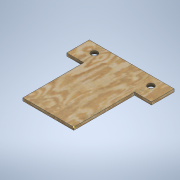
# Autodesk Inventor part: shooter bottom
Saved by Autodesk Inventor 2020 (Build 240168000, 168)
## iProperties
Created: 2020-01-27
Part Number: shooter bottom
Material: Wood (Oak)
Document SubType Name: Modeling
Designer: 1cikaychapman
Density: 0.76 g/cm^3
Appearance: Plywood - Weathered
Author: 1cikaychapman
Autodesk Inventor part; units mm, degrees
ref_plane "YZ Plane" through (0, 0, 0) normal (1, 0, 0) x (0, 1, 0)
ref_plane "XZ Plane" through (0, 0, 0) normal (0, 1, 0) x (-1, 0, 0)
ref_plane "XY Plane" through (0, 0, 0) normal (0, 0, 1) x (1, 0, 0)
sketch "Sketch1" plane through (0, 0, 0) normal (0, 1, 0) x (-1, 0, 0)
  line L0 (228.6, 0) -> (228.6, -273.05)
  line L1 (0, -273.05) -> (0, 0)
  line L2 (0, 0) -> (-76.2, 0)
  line L3 (0, 0) -> (-76.2, 0)
  line L4 (228.6, 0) -> (0, 0)
  line L5 (228.6, -273.05) -> (304.8, -273.05)
  line L6 (304.8, -273.05) -> (304.8, -374.65)
  line L7 (304.8, -374.65) -> (-76.2, -374.65)
  line L8 (-76.2, -374.65) -> (-76.2, -273.05)
  line L9 (-76.2, -273.05) -> (0, -273.05)
  line L10 (114.3, -511.2369) -> (114.3, 135.5146) construction
  point P0 (304.8, 0)
  dimension "d1" = 273.05
  dimension "d8" = 228.6
  dimension "d9" = 76.2
  dimension "d10" = 76.2
  dimension "d11" = 101.6
  constraints: 22 end point, 4 perpendicular, 2 horizontal, 1 collinear, 1 parallel, 1 point on line, 1 vertical
  measures "d1" distance of L0.start L0.end
  measures "d8" distance of L1.end L0.start
  measures "d9" distance of L8.end L1.start
  measures "d10" distance of L0.end L5.end
  measures "d11" distance of L8.end L7.end
extrude "Extrusion1" add sketch "Sketch1" along normal blind 12.7
sketch "Sketch2" plane through (0, 12.7, 0) normal (0, 1, 0) x (1, 0, 0)
  point P0 (0, 0)
sketch "Sketch3" plane through (0, 12.7, 0) normal (0, 1, 0) x (1, 0, 0)
  line L0 (-114.3, 418.531) -> (-114.3, -18.8119) construction
  circle A0 centre (-241.3, 334.01) radius 14.2875
  line L1 (-304.8, 273.05) -> (-228.6, 273.05) construction
  line L2 (0, 273.05) -> (76.2, 273.05) construction
  circle A1 centre (12.7, 334.01) radius 14.2875
  point P0 (0, 0)
  dimension "d19" = 114.3
  dimension "d20" = 28.575
  dimension "d23" = 60.96
  dimension "d26" = 127
  dimension "d27" = 28.575
  dimension "d28" = 60.96
  dimension "d29" = 127
  constraints: 2 centre point, 2 end point, 1 vertical
  measures "d19" horizontal distance of point (0, 0) L0.end
  measures "d20" diameter of A0
  measures "d23" distance from line of L1 A0.centre
  measures "d26" distance from line of L0 A0.centre
  measures "d27" diameter of A1
  measures "d28" vertical distance of L2.end A1.centre
  measures "d29" distance from line of L0 A1.centre
extrude "Extrusion2" cut sketch "Sketch3" against normal through all
body "Solid1"
